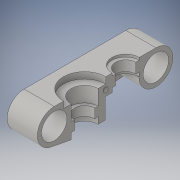
# Autodesk Inventor part: Hotend holder V4
Saved by Autodesk Inventor 2016 (Build 200138000, 138)
## iProperties
Created: 2016-02-11
Part Number: Hotend holder V4
Material: Generic
Document SubType Name: Modeling
Designer: Scott
Density: 1 g/cm^3
Appearance: Default
Author: Scott
Autodesk Inventor part; units mm, degrees
ref_plane "YZ Plane" through (0, 0, 0) normal (1, 0, 0) x (0, 1, 0)
ref_plane "XZ Plane" through (0, 0, 0) normal (0, 1, 0) x (-1, 0, 0)
ref_plane "XY Plane" through (0, 0, 0) normal (0, 0, 1) x (1, 0, 0)
sketch "Sketch1" plane through (0, 0, 0) normal (1, 0, 0) x (0, 1, 0)
  line L0 (0, 0) -> (0, -68)
  line L1 (0, -68) -> (0, -60)
  line L2 (0, 0) -> (0, -8)
  circle A0 centre (0, -4) radius 4
  circle A1 centre (0, -64) radius 4
  circle A2 centre (0, -64) radius 7.5
  circle A3 centre (0, -4) radius 7.5
  circle A4 centre (0, -4) radius 10
  circle A5 centre (0, -64) radius 10
  line L3 (10, -4) -> (10, -64)
  dimension "d5" = 20
  dimension "d6" = 20
  dimension "d0" = 68
  dimension "d1" = 8
  dimension "d2" = 8
  dimension "d3" = 15
  dimension "d4" = 15
  constraints: 8 end point, 4 coincident, 2 centre point, 2 horizontal alignment, 2 midpoint, 2 point on line, 2 vertical, 2 vertical alignment, 8 other
  measures "d0" distance of L0.start L0.end
  measures "d1" distance of L0.end L1.end
  measures "d2" distance of L0.start L2.end
  measures "d3" diameter of A2
  measures "d4" diameter of A3
extrude "Extrusion1" add sketch "Sketch1" along normal blind 15.24 contours A4 | A5
sketch "Sketch2" plane through (0, 0, -4) normal (-1, 0, 0) x (0, 0, 1)
  circle A0 centre (0, 0) radius 10 projected
  line L0 (0, 10) -> (-60, 10)
  circle A1 centre (-60, 0) radius 10 projected
  line L1 (-50, 0) -> (-10, 0)
  point P0 (4, 0)
  constraints: 4 end point, 4 point on circle, 1 parallel, 1 tangent
extrude "Extrusion2" add sketch "Sketch2" along normal blind 2.54
sketch "Sketch3" plane through (0, 0, -4) normal (1, 0, 0) x (0, 0, -1)
  line L0 (0, 10) -> (60, 10) projected
  arc A0 (10, 0) -> (0, 10) centre (0, 0) ccw projected
  line L1 (50, 0) -> (10, 0) projected
  arc A1 (60, 10) -> (50, 0) centre (60, 0) ccw projected
  line L2 (0, 10) -> (60, 10) projected
  point P0 (-4, 0)
extrude "Extrusion3" add sketch "Sketch3" along normal up to surface (15.24 mm away)
sketch "Sketch4" plane through (-2.54, 0, -14) normal (0, -1, 0) x (1, 0, 0)
  line L0 (0, 0) -> (17.78, 0) projected
  line L1 (17.78, 0) -> (17.78, -15.875)
  line L2 (17.78, -40) -> (0, -40) projected
  line L3 (17.78, -40) -> (17.78, 0) projected
  arc A0 (17.78, -24.125) -> (17.78, -40.1897) centre (17.78, -32.1574) ccw
  line L4 (17.78, 0) -> (17.78, -15.875)
  arc A1 (17.78, 0) -> (17.78, -15.875) centre (17.78, -7.9375) ccw
  line L5 (17.78, -24.125) -> (17.78, -40.1897)
  point P0 (2.54, 14)
  dimension "d13" = 15.875
  dimension "d16" = 15.875
  constraints: 6 end point, 4 point on circle, 2 centre point, 2 collinear, 2 point on line, 1 midpoint
  measures "d13" distance of L0.end L1.end
  measures "d16" distance of L2.start L5.start
extrude "Extrusion4" cut sketch "Sketch4" against normal blind 2.54
sketch "Sketch5" plane through (-2.54, 2.54, -14) normal (0, -1, 0) x (1, 0, 0)
  line L0 (17.78, 0) -> (17.78, 20) projected
  line L1 (17.78, -24.125) -> (17.78, -15.875) projected
  arc A0 (17.78, 0) -> (17.78, -15.875) centre (17.78, -7.9375) ccw projected
  line L2 (0, 0) -> (17.78, 0) projected
  line L3 (0, -40) -> (0, 0) projected
  line L4 (16.0445, -40) -> (0, -40) projected
  arc A1 (17.78, -24.125) -> (16.0445, -40) centre (17.78, -32.1574) ccw projected
  line L5 (17.78, -24.125) -> (17.78, -15.875) projected
  line L6 (17.78, 0) -> (17.78, -15.875)
  line L7 (17.78, 10) -> (17.78, -50) projected
  line L8 (17.78, -60) -> (17.78, -40) projected
  line L9 (17.78, -24.125) -> (17.78, -40)
  circle A2 centre (17.78, -7.9375) radius 6
  circle A3 centre (17.78, -32.1574) radius 6
  point P0 (2.54, 14)
  dimension "d20" = 12
  dimension "d21" = 12
  constraints: 4 end point, 2 centre point, 2 coincident, 2 vertical, 1 other
  measures "d20" diameter of A2
  measures "d21" diameter of A3
extrude "Extrusion5" cut sketch "Sketch5" against normal blind 6 contours A2 L6 | L6 A2 | A3 L7 | L7 A3
sketch "Sketch6" plane through (-2.54, 8.54, -14) normal (0, -1, 0) x (1, 0, 0)
  line L0 (17.78, -26.1574) -> (17.78, -38.1574) projected
  circle A0 centre (17.78, -32.1574) radius 8.0324
  line L1 (17.78, -1.9375) -> (17.78, -13.9375) projected
  arc A1 (17.78, -1.9375) -> (17.78, -13.9375) centre (17.78, -7.9375) ccw projected
  circle A2 centre (17.78, -7.9375) radius 7.9375
  point P0 (2.54, 14)
  constraints: 2 centre point, 1 coincident, 1 midpoint
extrude "Extrusion6" cut sketch "Sketch6" against normal blind 6 contours A0 | L1 A1 | A2
sketch "Sketch7" plane through (15.24, 0, 0) normal (1, 0, 0) x (0, 0, -1)
  line L0 (29.875, 10) -> (38.125, 10) projected
  arc A0 (4, 10) -> (14, 0) centre (4, 0) ccw projected
  line L1 (34, 10) -> (14, 10)
  line L2 (14, 10) -> (14, 0)
  line L3 (14, 0) -> (34, 0)
  line L4 (34, 0) -> (34, 10)
  point P0 (0, 0)
  constraints: 8 end point, 2 parallel, 1 horizontal, 1 midpoint, 1 perpendicular
extrude "Extrusion7" add sketch "Sketch7" against normal blind 12
sketch "Sketch8" plane through (15.24, 0, 0) normal (1, 0, 0) x (0, 0, -1)
  line L0 (54, 0) -> (14, 0) projected
  line L1 (34, 0) -> (14, 0)
  line L2 (14, 0) -> (14, -12.065)
  line L3 (14, -12.065) -> (34, -12.065)
  line L4 (34, -12.065) -> (34, 0)
  point P0 (0, 0)
  dimension "d28" = 12.065
  constraints: 8 end point, 2 parallel, 1 horizontal, 1 midpoint, 1 perpendicular
  measures "d28" distance of L2.end L1.end
extrude "Extrusion8" add sketch "Sketch8" against normal up to surface (17.78 mm away)
sketch "Sketch9" plane through (15.24, -12.065, -34) normal (0, -1, 0) x (1, 0, 0)
  line L0 (-17.78, 20) -> (0, 20) projected
  line L1 (0, 20) -> (0, 4.125)
  line L2 (0, 20) -> (0, 0) projected
  arc A0 (0, 20) -> (0, 4.125) centre (0, 12.0625) ccw
  point P0 (-15.24, 34)
  dimension "d31" = 15.875
  dimension "d32" = 7.9375
  constraints: 2 end point, 2 point on circle, 1 centre point
  measures "d31" distance of L0.end L1.end
  measures "d32" radius of A0
extrude "Extrusion9" cut sketch "Sketch9" against normal blind 3.81
sketch "Sketch10" plane through (15.24, -8.255, -34) normal (0, -1, 0) x (1, 0, 0)
  line L0 (0, 20) -> (0, 4.125) projected
  arc A0 (0, 20) -> (0, 4.125) centre (0, 12.0625) ccw projected
  circle A1 centre (0, 12.0625) radius 6
  point P0 (-15.24, 34)
  dimension "d35" = 12
  constraints: 1 centre point, 1 coincident
  measures "d35" diameter of A1
extrude "Extrusion10" cut sketch "Sketch10" against normal blind 5.5 contours A1 L0 | L0 A1
sketch "Sketch11" plane through (15.24, -2.755, -34) normal (0, -1, 0) x (1, 0, 0)
  line L0 (0, 18.0625) -> (0, 6.0625) projected
  circle A0 centre (0, 12.0625) radius 7.9375
  point P0 (-15.24, 34)
  constraints: 1 centre point, 1 midpoint
extrude "Extrusion11" cut sketch "Sketch11" against normal blind 9
sketch "Sketch12" plane through (15.24, 6.245, -34) normal (0, -1, 0) x (1, 0, 0)
  line L0 (0, 20) -> (0, 4.125) projected
  circle A0 centre (0, 12.0625) radius 12.5
  point P0 (-15.24, 34)
  dimension "d40" = 25
  constraints: 1 centre point, 1 midpoint
  measures "d40" diameter of A0
extrude "Extrusion12" cut sketch "Sketch12" against normal blind 9
sketch "Sketch13" plane through (15.24, 0, 0) normal (1, 0, 0) x (0, 0, -1)
  line L0 (9.4375, 6.245) -> (9.4375, 10) projected
  line L1 (4, 10) -> (9.4375, 10) projected
  arc A0 (4, 10) -> (14, 0) centre (4, 0) ccw projected
  line L2 (14, 0) -> (14, 6.245) projected
  line L3 (14, 6.245) -> (9.4375, 6.245) projected
  circle A1 centre (4, 0) radius 7.5 projected
  line L4 (14, -8.255) -> (14, -12.065) projected
  line L5 (14, -12.065) -> (2.7589, -9.9227)
  arc A2 (4, 10) -> (14, 0) centre (4, 0) ccw projected
  line L6 (14, 0) -> (14, -12.065)
  line L7 (14, -12.065) -> (14, 0) projected
  line L8 (14, -12.065) -> (14, 0)
  line L9 (14, 0) -> (8.3795, -7.0711)
  line L10 (8.3795, -7.0711) -> (2.7589, -9.9227)
  point P0 (0, 0)
  constraints: 10 end point, 2 point on circle, 2 tangent, 1 collinear, 1 vertical
extrude "Extrusion13" add sketch "Sketch13" against normal up to surface (17.78 mm away) contours L6 L4 L5 A0
sketch "Sketch14" plane through (-2.54, 0, -4) normal (-1, 0, 0) x (0, 0, 1)
  line L0 (-30, -12.065) -> (-10, -12.065) projected
  arc A0 (1.2411, -9.9227) -> (0, 10) centre (0, 0) ccw projected
  arc A1 (1.2411, -9.9227) -> (0, 10) centre (0, 0) ccw projected
  line L1 (0, 10) -> (-60, 10) projected
  arc A2 (-60, 10) -> (-50, 0) centre (-60, 0) ccw projected
  line L2 (-50, 0) -> (-30, 0) projected
  line L3 (-30, 0) -> (-30, -12.065) projected
  line L4 (-30, -12.065) -> (-10, -12.065) projected
  line L5 (-10, -12.065) -> (1.2411, -9.9227) projected
  line L6 (-30, -12.065) -> (-58.9174, -9.9412)
  arc A3 (-60, 10) -> (-50, 0) centre (-60, 0) ccw projected
  point P0 (4, 0)
  constraints: 2 end point, 2 point on circle
extrude "Extrusion14" add sketch "Sketch14" against normal blind 2.54 contours L6 A2 L2 L3
sketch "Sketch15" plane through (0, 0, -4) normal (1, 0, 0) x (0, 0, -1)
  circle A0 centre (0, 0) radius 4.5
  circle A1 centre (60, 0) radius 7.5 projected
  circle A2 centre (60, 0) radius 4.5
  point P0 (-4, 0)
  dimension "d47" = 9
  dimension "d48" = 9
  constraints: 2 centre point, 1 coincident
  measures "d47" diameter of A0
  measures "d48" diameter of A2
extrude "Extrusion15" cut sketch "Sketch15" against normal blind 2.54 contours A0 | A2
sketch "Sketch16" plane through (15.24, 0, 0) normal (1, 0, 0) x (0, 0, -1)
  circle A0 centre (34.2867, 3.4117) radius 1.5
  point P0 (0, 0)
  dimension "d51" = 3
  constraints: 1 centre point
  measures "d51" diameter of A0
extrude "Extrusion16" cut sketch "Sketch16" against normal blind 70.8025
body "Solid1"
